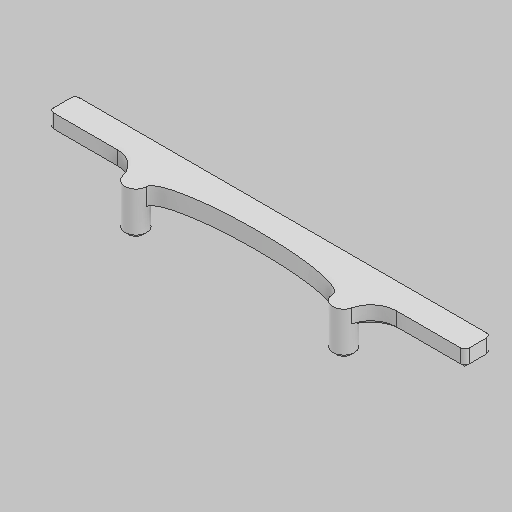
# Autodesk Inventor part: bumper
Saved by Autodesk Inventor 2026 (Build 300175000, 175)
## iProperties
Created: 2026-07-11
Part Number: bumper
Material: Generic
Document SubType Name: Modeling
Designer: admin
Density: 1 g/cm^3
Appearance: Default
Author: admin
Autodesk Inventor part; units mm, degrees
ref_plane "YZ Plane" through (0, 0, 0) normal (1, 0, 0) x (0, 1, 0)
ref_plane "XZ Plane" through (0, 0, 0) normal (0, 1, 0) x (-1, 0, 0)
ref_plane "XY Plane" through (0, 0, 0) normal (0, 0, 1) x (1, 0, 0)
sketch "Эскиз1" plane through (0, 0, 0) normal (0, 1, 0) x (-1, 0, 0)
  line L0 (0, -2) -> (0, 4)
  circle A0 centre (24, 8) radius 2.5
  ellipse E0 centre (0, 8) end of major axis (21.5, 8) minor radius 4
  line L1 (0, -2) -> (48, -2)
  line L2 (48, -2) -> (48, 4)
  line L3 (48, 4) -> (32.2614, 4)
  arc A1 (26.4298, 8.5882) -> (32.2614, 4) centre (32.2614, 10) ccw
  point P0 (0, 0)
  point P1 (0, 1)
  point P2 (26.5, 8)
  point P3 (21.5, 8)
  dimension "d0" = 5
  dimension "d1" = 48
  dimension "d2" = 8
  dimension "d14" = 4
  dimension "d15" = 2
  dimension "d16" = 48
  dimension "d17" = 6
  dimension "d18" = 6
  constraints: 8 end point, 4 point on circle, 2 centre point, 2 horizontal alignment, 2 tangent, 2 vertical, 1 horizontal, 1 midpoint, 1 perpendicular, 1 point on line, 1 vertical alignment, 4 other
  measures "d0" diameter of A0
  measures "d1" diameter of A0.centre L0
  measures "d2" vertical distance of A0.centre point (0, 0)
  measures "d14" distance of point (0, 0) L0.end
  measures "d15" distance of L0.start point (0, 0)
  measures "d16" distance of L0.start L1.end
  measures "d17" distance between parallel lines of L1 L3
  measures "d18" radius of A1
extrude "Выдавливание1" add sketch "Эскиз1" along normal blind 4 contours L0 E0 A0 A1 L3 L2 L1 | A0
extrude "Выдавливание2" add sketch "Эскиз1" against normal blind 6 contours A0
chamfer "Фаска3" distance 0.8 angle 45 1 edges at (-21.5, -6, 8)
fillet "Сопряжение1" radius 1 2 edges at (-48, 2, -2) (-48, 2, 4)
chamfer "Фаска4" distance 0.8 angle 45 6 edges at (-23.5, 0, -2) (-47.7071, 0, -1.7071) (-48, 0, 1) (-47.7071, 0, 3.7071) (-39.6307, 0, 4) (-28.5513, 0, 5.2846)
mirror "Зеркальное отражение1" about plane through (0, 0, 4) normal (1, 0, 0)
